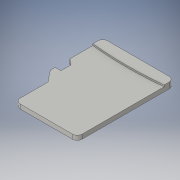
# Autodesk Inventor part: MicroSD Card
Saved by Autodesk Inventor 2016 (Build 200138000, 138)
## iProperties
Created: 2015-11-27
Part Number: MicroSD Card
Material: Generic
Document SubType Name: Modeling
Designer: Spooner
Density: 1 g/cm^3
Appearance: Default
Author: Spooner
Autodesk Inventor part; units mm, degrees
ref_plane "YZ Plane" through (0, 0, 0) normal (1, 0, 0) x (0, 1, 0)
ref_plane "XZ Plane" through (0, 0, 0) normal (0, 1, 0) x (-1, 0, 0)
ref_plane "XY Plane" through (0, 0, 0) normal (0, 0, 1) x (1, 0, 0)
sketch "Sketch1" plane through (0, 0, 0) normal (0, 1, 0) x (-1, 0, 0)
  line L0 (-1.4224, 0) -> (-11.049, 0)
  line L1 (-11.049, 0) -> (-11.049, -14.986)
  line L2 (-11.049, -14.986) -> (0, -14.986)
  line L3 (0, -14.986) -> (0, -9.906)
  line L4 (0, -9.906) -> (-0.889, -9.144)
  line L5 (-0.889, -9.144) -> (-0.889, -7.62)
  line L6 (-0.889, -7.62) -> (0, -7.62)
  line L7 (0, -7.62) -> (0, -6.858)
  line L8 (0, -6.858) -> (-1.4224, -5.08)
  line L9 (-1.4224, -5.08) -> (-1.4224, 0)
  point P0 (0, 0)
  dimension "d0" = 14.986
  dimension "d1" = 11.049
  dimension "d2" = 9.6266
  dimension "d3" = 0.889
  dimension "d4" = 5.08
  dimension "d5" = 7.62
  dimension "d6" = 0.762
  dimension "d7" = 1.778
  dimension "d8" = 5.08
  constraints: 20 end point, 5 perpendicular, 2 point on line, 1 horizontal, 1 horizontal alignment, 1 parallel, 1 vertical alignment
  measures "d0" distance of L0.end L1.end
  measures "d1" distance of L1.end L2.end
  measures "d2" distance of L0.start L0.end
  measures "d3" distance from line of L3 L4.end
  measures "d4" distance of L2.end L3.end
  measures "d5" vertical distance of L0.start L6.end
  measures "d6" vertical distance of L3.end L4.end
  measures "d7" vertical distance of L8.end L7.end
  measures "d8" distance of L8.end L0.start
extrude "Extrusion1" add sketch "Sketch1" along normal blind 0.6858
fillet "Fillet1" radius 0.762 4 edges at (11.049, 0.3429, -14.986) (0, 0.3429, -14.986) (11.049, 0.3429, 0) (1.4224, 0.3429, 0)
sketch "Sketch2" plane through (0, 0.6858, 0) normal (0, 1, 0) x (1, 0, 0)
  arc A0 (1.4224, 0.762) -> (2.1844, 0) centre (2.1844, 0.762) ccw projected
  line L0 (2.1844, 0) -> (10.287, 0) projected
  arc A1 (10.287, 0) -> (11.049, 0.762) centre (10.287, 0.762) ccw projected
  line L1 (11.049, 0.762) -> (11.049, 14.224) projected
  arc A2 (11.049, 14.224) -> (10.287, 14.986) centre (10.287, 14.224) ccw projected
  line L2 (10.287, 14.986) -> (0.762, 14.986) projected
  arc A3 (0.762, 14.986) -> (0, 14.224) centre (0.762, 14.224) ccw projected
  line L3 (0, 14.224) -> (0, 9.906) projected
  line L4 (0, 9.906) -> (0.889, 9.144) projected
  line L5 (0.889, 9.144) -> (0.889, 7.62) projected
  line L6 (0.889, 7.62) -> (0, 7.62) projected
  line L7 (0, 7.62) -> (0, 6.858) projected
  line L8 (0, 6.858) -> (1.4224, 5.08) projected
  line L9 (1.4224, 5.08) -> (1.4224, 0.762) projected
  line L10 (0, 14.224) -> (0, 9.906) projected
  arc A4 (0, 13.462) -> (11.049, 13.462) centre (5.5245, 65.5585) ccw
  point P0 (0, 0)
  dimension "d12" = 1.524
  dimension "d13" = 1.8161
  constraints: 2 point on circle, 2 point on line, 1 centre point, 1 horizontal alignment
  measures "d12" distance from line of L2 A4.start
  measures "d13" distance edge to line of A4 L2
extrude "Extrusion2" add sketch "Sketch2" along normal blind 0.254 contours A4 L3 A3 L2 A2 L1
body "Solid1"
